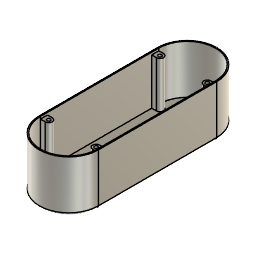
TRARM02_Link2B_100x50x43 (Autodesk Fusion 360 design; units mm, degrees)
Autodesk Fusion 360 part; units mm, degrees
note: some values were not read from the file. Set by a fixed rule: which sketch regions a step uses.
sketch "스케치1" plane through (0, 0, 0) normal (0, 0, 1) x (1, 0, 0)
  line L0 (25, 100) -> (25, 0)
  line L1 (-25, 100) -> (-25, 0)
  arc A0 (25, 100) -> (-25, 100) centre (0, 100) ccw
  arc A1 (-25, 0) -> (25, 0) centre (0, 0) ccw
  dimension "d1" = 50
  dimension "d140" = 100
  constraint coincident A1.centre origin
  constraint vertical A1.centre A0.centre
  constraint vertical L0
  constraint tangent L1 A0
  constraint parallel L0 L1
  constraint horizontal A1.centre L1.end
  constraint horizontal A1.centre L0.end
  measures "d1" diameter of A1
  measures "d140" distance of L1.start L1.end
extrude "돌출1" add sketch "스케치1" along normal blind 2
sketch "스케치2" plane through (0, 0, 2) normal (0, 0, 1) x (-1, 0, 0)
  arc A0 (-25, -100) -> (25, -100) centre (0, -100) ccw
  line L0 (25, -100) -> (25, 0)
  arc A1 (25, 0) -> (-25, 0) centre (0, 0) ccw
  line L1 (-25, 0) -> (-25, -100)
  line L2 (-24, -6) -> (-24, -94)
  line L3 (-20, -6) -> (-24, -6)
  arc A2 (-20, -6) -> (-20, 0) centre (-20, -3) ccw
  line L4 (20, -6) -> (24, -6)
  line L5 (20, 0) -> (24, 0)
  line L6 (24, -94) -> (24, -6)
  arc A3 (20, 0) -> (20, -6) centre (20, -3) ccw
  line L7 (-19.997, -94) -> (-24, -94)
  line L8 (19.997, -94) -> (24, -94)
  arc A4 (20.003, -94) -> (20, -100) centre (20, -97) ccw
  arc A5 (-19.997, -100) -> (-19.997, -94) centre (-20, -97) ccw
  arc A6 (-24, -100) -> (24, -100) centre (0, -100) ccw
  line L9 (-19.997, -100) -> (-24, -100)
  line L10 (20, -100) -> (24, -100)
  arc A7 (24, 0) -> (-24, 0) centre (0, 0) ccw
  line L11 (-20, 0) -> (-24, 0)
  dimension "d206" = 6
  dimension "d207" = 3
  dimension "d208" = 20
  dimension "d209" = 20
  dimension "d211" = 3
  constraint equal A2 A3
  constraint equal A2 A5
  constraint equal A4 A5
  constraint horizontal A2.centre A3.centre
  constraint horizontal A4.centre A5.centre
  constraint vertical A5.centre A2.centre
  constraint vertical A4.centre A3.centre
  constraint horizontal L3
  constraint perpendicular L4 L6
  constraint perpendicular L5 L6
  constraint equal L4 L5
  constraint coincident L7.start A5
  constraint perpendicular L2 L7
  constraint coincident L8.start A4
  constraint perpendicular L6 L8
  constraint coincident L8 A4.start
  constraint coincident L7 A5.end
  constraint equal L7 L8
  constraint concentric A0 A6
  constraint coincident L7.start A5.end
  constraint horizontal A6.start A5.start
  constraint horizontal A6.start A0.centre
  constraint vertical A5.start L7.start
  constraint tangent A4 L10
  constraint vertical L6.start A6.end
  constraint horizontal L10
  constraint concentric A1 A7
  constraint horizontal A1.end A7.end
  constraint vertical A2.centre A2.end
  constraint vertical A2.centre L3.start
  constraint horizontal L0.end L5.end
  constraint vertical A7.end L2.start
  measures "d206" diameter of A2
  measures "d207" vertical distance of A1.centre A2.centre
  measures "d208" horizontal distance of A1.centre A2.centre
  measures "d209" horizontal distance of A1.centre A3.centre
  measures "d211" vertical distance of A0.centre A5.centre
extrude "돌출25" add sketch "스케치2" along normal blind 41
sketch "스케치22" plane through (0, 0, 43) normal (0, 0, 1) x (-1, 0, 0)
  arc A0 (20, 0) -> (20, -6) centre (20, -3) ccw
  line L0 (20, -6) -> (24, -6)
  line L1 (24, 0) -> (20, 0)
  arc A1 (-20, -6) -> (-20, 0) centre (-20, -3) ccw
  line L2 (-24, -6) -> (-20, -6)
  line L3 (-19.997, -94) -> (-24, -94)
  arc A2 (-19.997, -100) -> (-19.997, -94) centre (-20, -97) ccw
  line L4 (24, -94) -> (20.003, -94)
  arc A3 (20.003, -94) -> (20, -100) centre (20, -97) ccw
  line L5 (24, -6) -> (24, 0)
  line L6 (20, -100) -> (24, -100)
  line L7 (24, -100) -> (24, -94)
  line L8 (-19.997, -100) -> (-24, -100)
  line L9 (-24, -100) -> (-24, -94)
  line L10 (-24, 0) -> (-20, 0)
  line L11 (-20, 0) -> (-24, 0)
  line L12 (-24, -6) -> (-24, 0)
  point P0 (24, -100)
  point P1 (-24, -100)
  point P2 (-24, 0)
  constraint coincident L0.end L5.start
  constraint coincident L1.start L5.end
  constraint coincident A3.end L6.start
  constraint coincident P0 L6.end
  constraint coincident L4.start L7.end
  constraint coincident A2.start L8.start
  constraint coincident P1 L8.end
  constraint coincident L3.end L9.end
  constraint coincident A1.end L10.end
  constraint coincident P2 L10.start
  constraint coincident L2.start L12.start
extrude "돌출26" cut sketch "스케치22" against normal blind 2
sketch "스케치23" plane through (0, 0, 41) normal (0, 0, 1) x (-1, 0, 0)
  circle A0 centre (20, -3) radius 1.45
  circle A1 centre (-20, -3) radius 1.45
  circle A2 centre (-20, -97) radius 1.45
  circle A3 centre (20, -97) radius 1.45
  arc A4 (-19.997, -100) -> (-19.997, -94) centre (-20, -97) ccw
  arc A5 (20.003, -94) -> (20, -100) centre (20, -97) ccw
  arc A6 (20, 0) -> (20, -6) centre (20, -3) ccw
  arc A7 (-20, -6) -> (-20, 0) centre (-20, -3) ccw
  dimension "d217" = 2.9
  constraint equal A2 A3
  constraint equal A1 A2
  constraint equal A0 A1
  constraint concentric A2 A4
  constraint concentric A3 A5
  constraint concentric A0 A6
  constraint concentric A1 A7
  measures "d217" diameter of A1
extrude "돌출27" cut sketch "스케치23" against normal blind 5
fillet "필렛5" radius 2 4 edges at (0, -25, 0) (-25, 50, 0) (0, 125, 0) (25, 50, 0)
